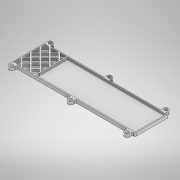
# Autodesk Inventor part: backtpackCOVER2
Saved by Autodesk Inventor 2021 (Build 250183000, 183)
## iProperties
Created: 2021-09-03
Part Number: backtpackCOVER2
Material: Generic
Document SubType Name: Modeling
Designer: perez
Density: 1 g/cm^3
Appearance: Default
Author: perez
Autodesk Inventor part; units mm, degrees
ref_plane "YZ Plane" through (0, 0, 0) normal (1, 0, 0) x (0, 1, 0)
ref_plane "XZ Plane" through (0, 0, 0) normal (0, 1, 0) x (-1, 0, 0)
ref_plane "XY Plane" through (0, 0, 0) normal (0, 0, 1) x (1, 0, 0)
sketch "Sketch1" plane through (0, 0, 0) normal (0, 1, 0) x (-1, 0, 0)
  line L0 (0, 0) -> (37, 0) construction
  line L1 (37, 0) -> (37, -30) construction
  line L2 (37, -30) -> (0, -30) construction
  line L3 (0, -30) -> (0, 0) construction
  line L4 (75.5, -6) -> (38, -6) construction
  line L5 (38, -6) -> (38, -24) construction
  line L6 (38, -24) -> (75.5, -24) construction
  line L7 (75.5, -24) -> (75.5, -6) construction
  line L8 (94, 0) -> (76.5, 0) construction
  line L9 (76.5, 0) -> (76.5, -28) construction
  line L10 (76.5, -28) -> (94, -28) construction
  line L11 (94, -28) -> (94, 0) construction
  line L12 (-1, 1) -> (117.5, 1)
  line L13 (117.5, 1) -> (117.5, -31)
  line L14 (117.5, -31) -> (-1, -31)
  line L15 (-1, -31) -> (-1, 1)
  line L16 (0, 0) -> (94, 0)
  line L17 (94, 0) -> (94, -30)
  line L18 (94, -30) -> (0, -30)
  line L19 (0, -30) -> (0, 0)
  line L20 (38, -8) -> (37, -8)
  line L21 (37, -8) -> (37, -22)
  line L22 (37, -22) -> (38, -22)
  line L23 (38, -22) -> (38, -8)
  line L24 (73.5, -6) -> (40, -6)
  line L25 (40, -6) -> (40, -5)
  line L26 (40, -5) -> (73.5, -5)
  line L27 (73.5, -5) -> (73.5, -6)
  line L28 (73.5, -24) -> (40, -24)
  line L29 (40, -24) -> (40, -25)
  line L30 (40, -25) -> (73.5, -25)
  line L31 (73.5, -25) -> (73.5, -24)
  line L32 (76.5, -8) -> (75.5, -8)
  line L33 (75.5, -8) -> (75.5, -22)
  line L34 (75.5, -22) -> (76.5, -22)
  line L35 (76.5, -22) -> (76.5, -8)
  line L36 (115, -31) -> (115, -33.5) construction
  line L37 (58.25, -31) -> (58.25, -33.5) construction
  line L38 (4, -31) -> (4, -33.5) construction
  line L39 (115, 1) -> (115, 3.5) construction
  line L40 (58.25, 1) -> (58.25, 3.5) construction
  line L41 (4, 1) -> (4, 3.5) construction
  circle A0 centre (115, -33.5) radius 2.5
  circle A1 centre (58.25, -33.5) radius 2.5
  circle A2 centre (4, -33.5) radius 2.5
  circle A3 centre (4, 3.5) radius 2.5
  circle A4 centre (58.25, 3.5) radius 2.5
  circle A5 centre (115, 3.5) radius 2.5
  line L42 (117.5, 1) -> (117.5, 3.5)
  line L43 (112.5, 3.5) -> (112.5, 1)
  line L44 (60.75, 3.5) -> (60.75, 1)
  line L45 (55.75, 3.5) -> (55.75, 1)
  line L46 (6.5, 3.5) -> (6.5, 1)
  line L47 (1.5, 3.5) -> (1.5, 1)
  line L48 (1.5, -33.5) -> (1.5, -31)
  line L49 (6.5, -33.5) -> (6.5, -31)
  line L50 (55.75, -33.5) -> (55.75, -31)
  line L51 (60.75, -33.5) -> (60.75, -31)
  line L52 (117.5, -33.5) -> (117.5, -31)
  line L53 (112.5, -33.5) -> (112.5, -31)
  circle A6 centre (115, -33.5) radius 1.55
  circle A7 centre (58.25, -33.5) radius 1.55
  circle A8 centre (4, -33.5) radius 1.55
  circle A9 centre (4, 3.5) radius 1.55
  circle A10 centre (58.25, 3.5) radius 1.55
  circle A11 centre (115, 3.5) radius 1.55
  line L54 (57.75, -30) -> (58.75, -30)
  line L55 (58.75, -30) -> (58.75, -25)
  line L56 (58.75, -25) -> (57.75, -25)
  line L57 (57.75, -25) -> (57.75, -30)
  line L58 (57.75, -5) -> (58.75, -5)
  line L59 (58.75, -5) -> (58.75, 0)
  line L60 (58.75, 0) -> (57.75, 0)
  line L61 (57.75, 0) -> (57.75, -5)
  line L62 (40, -25) -> (41, -25)
  line L63 (41, -25) -> (41, -30)
  line L64 (41, -30) -> (40, -30)
  line L65 (40, -30) -> (40, -25)
  line L66 (40, -5) -> (41, -5)
  line L67 (41, -5) -> (41, 0)
  line L68 (41, 0) -> (40, 0)
  line L69 (40, 0) -> (40, -5)
  line L70 (73.5, -5) -> (72.5, -5)
  line L71 (72.5, -5) -> (72.5, 0)
  line L72 (72.5, 0) -> (73.5, 0)
  line L73 (73.5, 0) -> (73.5, -5)
  line L74 (73.5, -25) -> (72.5, -25)
  line L75 (72.5, -25) -> (72.5, -30)
  line L76 (72.5, -30) -> (73.5, -30)
  line L77 (73.5, -30) -> (73.5, -25)
  dimension "d0" = 37
  dimension "d1" = 30
  dimension "d2" = 18
  dimension "d3" = 37.5
  dimension "d4" = 1
  dimension "d5" = 6
  dimension "d6" = 17.5
  dimension "d7" = 28
  dimension "d8" = 1
  dimension "d9" = 1
  dimension "d10" = 1
  dimension "d11" = 1
  dimension "d12" = 117.5
  dimension "d13" = 2
  dimension "d14" = 2
  dimension "d15" = 1
  dimension "d16" = 1
  dimension "d17" = 2
  dimension "d18" = 2
  dimension "d19" = 2
  dimension "d20" = 2
  dimension "d21" = 2.5
  dimension "d22" = 2.5
  dimension "d23" = 5
  dimension "d24" = 2.5
  dimension "d25" = 2.5
  dimension "d26" = 2.5
  dimension "d27" = 2.5
  dimension "d28" = 5
  dimension "d29" = 5
  dimension "d30" = 2.5
  dimension "d31" = 3.1
  dimension "d32" = 3.1
  dimension "d33" = 3.1
  dimension "d34" = 3.1
  dimension "d35" = 3.1
  dimension "d36" = 3.1
  dimension "d44" = 1
  dimension "d45" = 1
  dimension "d46" = 0.5
  dimension "d47" = 0
  dimension "d48" = 1
  dimension "d49" = 1
  dimension "d50" = 1
  dimension "d51" = 1
  constraints: 152 end point, 30 parallel, 24 point on line, 16 point on circle, 15 perpendicular, 14 horizontal, 12 centre point, 12 coincident, 12 vertical, 8 tangent, 22 other
  measures "d0" distance of L1.end L2.end
  measures "d1" distance of L0.end L1.end
  measures "d2" distance of L4.end L5.end
  measures "d3" distance of L5.end L6.end
  measures "d4" distance between parallel lines of L1 L5
  measures "d5" distance between parallel lines of L2 L6
  measures "d6" distance of L10.end L9.end
  measures "d7" distance of L9.end L8.end
  measures "d8" distance between parallel lines of L7 L9
  measures "d9" distance between parallel lines of L15 L3
  measures "d12" distance between parallel lines of L13 L3
  measures "d13" distance between parallel lines of L20 L4
  measures "d14" distance between parallel lines of L22 L6
  measures "d15" distance of L30.end L28.start
  measures "d16" distance of L26.end L24.start
  measures "d17" distance between parallel lines of L5 L25
  measures "d18" distance between parallel lines of L7 L27
  measures "d19" distance between parallel lines of L6 L34
  measures "d20" distance between parallel lines of L4 L32
  measures "d21" distance of L36.start L36.end
  measures "d22" distance between parallel lines of L13 L36
  measures "d23" distance between parallel lines of L15 L38
  measures "d24" distance of L37.start L37.end
  measures "d25" distance of L39.start L39.end
  measures "d26" distance of L40.start L40.end
  measures "d27" distance of L41.start L41.end
  measures "d28" diameter of A0
  measures "d29" diameter of A1
  measures "d30" distance of L38.start L38.end
  measures "d31" diameter of A6
  measures "d32" diameter of A7
  measures "d33" diameter of A8
  measures "d34" diameter of A9
  measures "d35" diameter of A10
  measures "d36" diameter of A11
  measures "d44" distance between parallel lines of L55 L57
  measures "d45" distance between parallel lines of L59 L61
  measures "d46" distance between parallel lines of L37 L57
  measures "d47" distance between parallel lines of L40 L37
  measures "d48" distance of L63.end L64.end
  measures "d49" distance of L68.end L67.end
  measures "d50" distance of L71.end L72.end
  measures "d51" distance of L76.end L75.end
extrude "Extrusion1" add sketch "Sketch1" along normal blind 7 contours L12 L13 L14 L15 | L47 A3 L12 | A3 L46 L12 | A3 | L14 A2 L48 | L14 L49 A2 | A2 | L45 A4 L12 | A4 L44 L12 | A4 | L14 A1 L50 | L14 L51 A1 | A1 | L43 A5 L12 | A5 L42 L12 | A5 | L14 A0 L53 | L14 L52 A0 | A0 | L16 L67 L26 L69 | L26 L27 L24 L25 | L65 L30 L63 L18 | L16 L59 L26 L61 | L29 L28 L31 L30 | L57 L30 L55 L18 | L16 L73 L26 L71 | L75 L30 L77 L18 | L23 L22 L21 L20 | L35 L34 L33 L32
sketch "Sketch2" plane through (0, 0, 0) normal (0, -1, 0) x (1, 0, 0)
  line L0 (-117.5, -33.5) -> (-117.5, 3.5) projected
  arc A0 (-117.5, -33.5) -> (-112.5, -33.5) centre (-115, -33.5) ccw projected
  line L1 (-112.5, -31) -> (-112.5, -33.5) projected
  line L2 (-60.75, -31) -> (-112.5, -31) projected
  line L3 (-60.75, -33.5) -> (-60.75, -31) projected
  arc A1 (-60.75, -33.5) -> (-55.75, -33.5) centre (-58.25, -33.5) ccw projected
  line L4 (-55.75, -31) -> (-55.75, -33.5) projected
  line L5 (-6.5, -31) -> (-55.75, -31) projected
  line L6 (-6.5, -33.5) -> (-6.5, -31) projected
  arc A2 (-6.5, -33.5) -> (-1.5, -33.5) centre (-4, -33.5) ccw projected
  line L7 (-1.5, -31) -> (-1.5, -33.5) projected
  line L8 (1, -31) -> (-1.5, -31) projected
  line L9 (1, 1) -> (1, -31) projected
  line L10 (-1.5, 1) -> (1, 1) projected
  line L11 (-1.5, 3.5) -> (-1.5, 1) projected
  arc A3 (-1.5, 3.5) -> (-6.5, 3.5) centre (-4, 3.5) ccw projected
  line L12 (-6.5, 1) -> (-6.5, 3.5) projected
  line L13 (-55.75, 1) -> (-6.5, 1) projected
  line L14 (-55.75, 3.5) -> (-55.75, 1) projected
  arc A4 (-55.75, 3.5) -> (-60.75, 3.5) centre (-58.25, 3.5) ccw projected
  line L15 (-60.75, 1) -> (-60.75, 3.5) projected
  line L16 (-112.5, 1) -> (-60.75, 1) projected
  line L17 (-112.5, 3.5) -> (-112.5, 1) projected
  arc A5 (-112.5, 3.5) -> (-117.5, 3.5) centre (-115, 3.5) ccw projected
  circle A6 centre (-58.25, 3.5) radius 1.55 projected
  circle A7 centre (-4, 3.5) radius 1.55 projected
  circle A8 centre (-4, -33.5) radius 1.55 projected
  circle A9 centre (-58.25, -33.5) radius 1.55 projected
  circle A10 centre (-115, 3.5) radius 1.55 projected
  circle A11 centre (-115, -33.5) radius 1.55 projected
  line L18 (-41, 0) -> (-57.75, 0) projected
  line L19 (0, -30) -> (0, 0) projected
  line L20 (-57.75, -30) -> (-41, -30) projected
  line L21 (-94, 0) -> (-94, -30) projected
  line L22 (-41, -5) -> (-41, 0) projected
  line L23 (-57.75, -5) -> (-41, -5) projected
  line L24 (-57.75, 0) -> (-57.75, -5) projected
  line L25 (-41, -30) -> (-41, -25) projected
  line L26 (-57.75, -25) -> (-57.75, -30) projected
  line L27 (-41, -25) -> (-57.75, -25) projected
  line L28 (-72.5, -25) -> (-72.5, -30) projected
  line L29 (-58.75, -25) -> (-72.5, -25) projected
  line L30 (-58.75, -30) -> (-58.75, -25) projected
  line L31 (-72.5, -30) -> (-58.75, -30) projected
  line L32 (-72.5, 0) -> (-72.5, -5) projected
  line L33 (-58.75, 0) -> (-72.5, 0) projected
  line L34 (-58.75, -5) -> (-58.75, 0) projected
  line L35 (-72.5, -5) -> (-58.75, -5) projected
  line L36 (-73.5, 0) -> (-94, 0) projected
  line L37 (-73.5, -6) -> (-73.5, 0) projected
  line L38 (-40, -6) -> (-73.5, -6) projected
  line L39 (-40, 0) -> (-40, -6) projected
  line L40 (0, 0) -> (-40, 0) projected
  line L41 (-40, -30) -> (0, -30) projected
  line L42 (-40, -24) -> (-40, -30) projected
  line L43 (-73.5, -24) -> (-40, -24) projected
  line L44 (-73.5, -30) -> (-73.5, -24) projected
  line L45 (-94, -30) -> (-73.5, -30) projected
extrude "Extrusion2" add sketch "Sketch2" along normal blind 1 contours L0 A5 L17 L16 L15 A4 L14 L13 L12 A3 L11 L10 L9 L8 L7 A2 L6 L5 L4 A1 L3 L2 L1 A0 | L22 L23 L24 L18 | L41 L42 L43 L44 L45 L21 L36 L37 L38 L39 L40 L19 | L26 L27 L25 L20 | L29 L30 L31 L28 | L33 L34 L35 L32
fillet "Fillet2" radius 1 32 edges at (-73.5, 3.5, -6) (-73.5, 3.5, -24) (-40, 3.5, -24) (1, 3, -31) (-1.5, 3, -31) (1, 3, 1) (-55.75, 3, -31) (-1.5, 3, 1) (-55.75, 3, 1) (-112.5, 3, 1) (-112.5, 3, -31) (-60.75, 3, -31) (-6.5, 3, -31) (-60.75, 3, 1) (-6.5, 3, 1) (-40, 3.5, -6) (-72.5, 3.5, 0) (-57.75, 3.5, 0) (-72.5, 3.5, -25) (-57.75, 3.5, -25) (-41, 3.5, -25) (-58.75, 3.5, -25) (-41, 3.5, 0) (-58.75, 3.5, 0) (-72.5, 3.5, -30) (-57.75, 3.5, -30) (-57.75, 3.5, -5) (-72.5, 3.5, -5) (-41, 3.5, -5) (-58.75, 3.5, -5) (-58.75, 3.5, -30) (-41, 3.5, -30)
sketch "Sketch5" plane through (0, 7, 0) normal (0, 1, 0) x (1, 0, 0)
  line L0 (-120.447, 38.9055) -> (3.6698, 38.9055)
  line L1 (3.6698, 38.9055) -> (3.6698, -10.7705)
  line L2 (3.6698, -10.7705) -> (-120.447, -10.7705)
  line L3 (-120.447, -10.7705) -> (-120.447, 38.9055)
  point P0 (0, 0)
  constraints: 8 end point, 2 parallel, 1 horizontal, 1 perpendicular
extrude "Extrusion5" cut sketch "Sketch5" against normal blind 7
sketch "Sketch14" plane through (0, 0, 0) normal (0, 1, 0) x (1, 0, 0)
  line L0 (0, 30) -> (-95, 30)
  line L1 (-95, 30) -> (-95, 0)
  line L2 (-95, 0) -> (0, 0)
  line L3 (0, 0) -> (0, 30)
  line L4 (-54.75, 31) -> (-7.5, 31) projected
  line L5 (1, 30) -> (1, 0) projected
  line L6 (-7.5, -1) -> (-54.75, -1) projected
  line L7 (-117.5, -3.5) -> (-117.5, 33.5) projected
  circle A0 centre (-58.25, -3.5) radius 1.55 projected
  circle A1 centre (-4, -3.5) radius 1.55 projected
  circle A2 centre (-4, 33.5) radius 1.55 projected
  circle A3 centre (-58.25, 33.5) radius 1.55 projected
  circle A4 centre (-115, -3.5) radius 1.55 projected
  circle A5 centre (-115, 33.5) radius 1.55 projected
  arc A6 (1, 30) -> (0, 31) centre (0, 30) ccw projected
  line L8 (-0.5, 31) -> (0, 31) projected
  arc A7 (-1.5, 32) -> (-0.5, 31) centre (-0.5, 32) ccw projected
  line L9 (-1.5, 33.5) -> (-1.5, 32) projected
  arc A8 (-1.5, 33.5) -> (-6.5, 33.5) centre (-4, 33.5) ccw projected
  line L10 (-6.5, 32) -> (-6.5, 33.5) projected
  arc A9 (-7.5, 31) -> (-6.5, 32) centre (-7.5, 32) ccw projected
  line L11 (-54.75, 31) -> (-7.5, 31) projected
  arc A10 (-55.75, 32) -> (-54.75, 31) centre (-54.75, 32) ccw projected
  line L12 (-55.75, 33.5) -> (-55.75, 32) projected
  arc A11 (-55.75, 33.5) -> (-60.75, 33.5) centre (-58.25, 33.5) ccw projected
  line L13 (-60.75, 32) -> (-60.75, 33.5) projected
  arc A12 (-61.75, 31) -> (-60.75, 32) centre (-61.75, 32) ccw projected
  line L14 (-111.5, 31) -> (-61.75, 31) projected
  arc A13 (-112.5, 32) -> (-111.5, 31) centre (-111.5, 32) ccw projected
  line L15 (-112.5, 33.5) -> (-112.5, 32) projected
  arc A14 (-112.5, 33.5) -> (-117.5, 33.5) centre (-115, 33.5) ccw projected
  line L16 (-117.5, -3.5) -> (-117.5, 33.5) projected
  arc A15 (-117.5, -3.5) -> (-112.5, -3.5) centre (-115, -3.5) ccw projected
  line L17 (-112.5, -2) -> (-112.5, -3.5) projected
  arc A16 (-111.5, -1) -> (-112.5, -2) centre (-111.5, -2) ccw projected
  line L18 (-61.75, -1) -> (-111.5, -1) projected
  arc A17 (-60.75, -2) -> (-61.75, -1) centre (-61.75, -2) ccw projected
  line L19 (-60.75, -3.5) -> (-60.75, -2) projected
  arc A18 (-60.75, -3.5) -> (-55.75, -3.5) centre (-58.25, -3.5) ccw projected
  line L20 (-55.75, -2) -> (-55.75, -3.5) projected
  arc A19 (-54.75, -1) -> (-55.75, -2) centre (-54.75, -2) ccw projected
  line L21 (-7.5, -1) -> (-54.75, -1) projected
  arc A20 (-6.5, -2) -> (-7.5, -1) centre (-7.5, -2) ccw projected
  line L22 (-6.5, -3.5) -> (-6.5, -2) projected
  arc A21 (-6.5, -3.5) -> (-1.5, -3.5) centre (-4, -3.5) ccw projected
  line L23 (-1.5, -2) -> (-1.5, -3.5) projected
  arc A22 (-0.5, -1) -> (-1.5, -2) centre (-0.5, -2) ccw projected
  line L24 (0, -1) -> (-0.5, -1) projected
  arc A23 (0, -1) -> (1, 0) centre (0, 0) ccw projected
  line L25 (1, 30) -> (1, 0) projected
  line L26 (-116.5, 0) -> (-96.2679, 0)
  line L27 (-96.2679, 0) -> (-96.2679, 30)
  line L28 (-96.2679, 30) -> (-116.5, 30)
  line L29 (-116.5, 30) -> (-116.5, 0)
  line L30 (-120.0355, 30) -> (-116.5, 33.5355)
  line L31 (-116.5, 33.5355) -> (-112.9645, 30)
  line L32 (-112.9645, 30) -> (-116.5, 26.4645)
  line L33 (-116.5, 26.4645) -> (-120.0355, 30)
  line L34 (-115.6376, 25.602) -> (-112.102, 22.0665)
  line L35 (-112.102, 22.0665) -> (-108.5665, 25.602)
  line L36 (-108.5665, 25.602) -> (-112.102, 29.1376)
  line L37 (-112.102, 29.1376) -> (-115.6376, 25.602)
  line L38 (-111.0355, 30) -> (-107.5, 33.5355)
  line L39 (-107.5, 26.4645) -> (-111.0355, 30)
  line L40 (-103.9645, 30) -> (-107.5, 26.4645)
  line L41 (-107.5, 33.5355) -> (-103.9645, 30)
  line L42 (-99.5665, 25.602) -> (-103.102, 29.1376)
  line L43 (-103.102, 29.1376) -> (-106.6376, 25.602)
  line L44 (-106.6376, 25.602) -> (-103.102, 22.0665)
  line L45 (-103.102, 22.0665) -> (-99.5665, 25.602)
  line L46 (-102.0355, 30) -> (-98.5, 33.5355)
  line L47 (-98.5, 26.4645) -> (-102.0355, 30)
  line L48 (-94.9645, 30) -> (-98.5, 26.4645)
  line L49 (-98.5, 33.5355) -> (-94.9645, 30)
  line L50 (-90.5665, 25.602) -> (-94.102, 29.1376)
  line L51 (-94.102, 29.1376) -> (-97.6376, 25.602)
  line L52 (-97.6376, 25.602) -> (-94.102, 22.0665)
  line L53 (-94.102, 22.0665) -> (-90.5665, 25.602)
  line L54 (-120.0355, 21) -> (-116.5, 24.5355)
  line L55 (-116.5, 17.4645) -> (-120.0355, 21)
  line L56 (-112.9645, 21) -> (-116.5, 17.4645)
  line L57 (-116.5, 24.5355) -> (-112.9645, 21)
  line L58 (-108.5665, 16.602) -> (-112.102, 20.1376)
  line L59 (-112.102, 20.1376) -> (-115.6376, 16.602)
  line L60 (-115.6376, 16.602) -> (-112.102, 13.0665)
  line L61 (-112.102, 13.0665) -> (-108.5665, 16.602)
  line L62 (-111.0355, 21) -> (-107.5, 24.5355)
  line L63 (-107.5, 17.4645) -> (-111.0355, 21)
  line L64 (-103.9645, 21) -> (-107.5, 17.4645)
  line L65 (-107.5, 24.5355) -> (-103.9645, 21)
  line L66 (-99.5665, 16.602) -> (-103.102, 20.1376)
  line L67 (-103.102, 20.1376) -> (-106.6376, 16.602)
  line L68 (-106.6376, 16.602) -> (-103.102, 13.0665)
  line L69 (-103.102, 13.0665) -> (-99.5665, 16.602)
  line L70 (-102.0355, 21) -> (-98.5, 24.5355)
  line L71 (-98.5, 17.4645) -> (-102.0355, 21)
  line L72 (-94.9645, 21) -> (-98.5, 17.4645)
  line L73 (-98.5, 24.5355) -> (-94.9645, 21)
  line L74 (-90.5665, 16.602) -> (-94.102, 20.1376)
  line L75 (-94.102, 20.1376) -> (-97.6376, 16.602)
  line L76 (-97.6376, 16.602) -> (-94.102, 13.0665)
  line L77 (-94.102, 13.0665) -> (-90.5665, 16.602)
  line L78 (-120.0355, 12) -> (-116.5, 15.5355)
  line L79 (-116.5, 8.4645) -> (-120.0355, 12)
  line L80 (-112.9645, 12) -> (-116.5, 8.4645)
  line L81 (-116.5, 15.5355) -> (-112.9645, 12)
  line L82 (-108.5665, 7.602) -> (-112.102, 11.1376)
  line L83 (-112.102, 11.1376) -> (-115.6376, 7.602)
  line L84 (-115.6376, 7.602) -> (-112.102, 4.0665)
  line L85 (-112.102, 4.0665) -> (-108.5665, 7.602)
  line L86 (-111.0355, 12) -> (-107.5, 15.5355)
  line L87 (-107.5, 8.4645) -> (-111.0355, 12)
  line L88 (-103.9645, 12) -> (-107.5, 8.4645)
  line L89 (-107.5, 15.5355) -> (-103.9645, 12)
  line L90 (-99.5665, 7.602) -> (-103.102, 11.1376)
  line L91 (-103.102, 11.1376) -> (-106.6376, 7.602)
  line L92 (-106.6376, 7.602) -> (-103.102, 4.0665)
  line L93 (-103.102, 4.0665) -> (-99.5665, 7.602)
  line L94 (-102.0355, 12) -> (-98.5, 15.5355)
  line L95 (-98.5, 8.4645) -> (-102.0355, 12)
  line L96 (-94.9645, 12) -> (-98.5, 8.4645)
  line L97 (-98.5, 15.5355) -> (-94.9645, 12)
  line L98 (-90.5665, 7.602) -> (-94.102, 11.1376)
  line L99 (-94.102, 11.1376) -> (-97.6376, 7.602)
  line L100 (-97.6376, 7.602) -> (-94.102, 4.0665)
  line L101 (-94.102, 4.0665) -> (-90.5665, 7.602)
  line L102 (-120.0355, 3) -> (-116.5, 6.5355)
  line L103 (-116.5, -0.5355) -> (-120.0355, 3)
  line L104 (-112.9645, 3) -> (-116.5, -0.5355)
  line L105 (-116.5, 6.5355) -> (-112.9645, 3)
  line L106 (-108.5665, -1.398) -> (-112.102, 2.1376)
  line L107 (-112.102, 2.1376) -> (-115.6376, -1.398)
  line L108 (-115.6376, -1.398) -> (-112.102, -4.9335)
  line L109 (-112.102, -4.9335) -> (-108.5665, -1.398)
  line L110 (-111.0355, 3) -> (-107.5, 6.5355)
  line L111 (-107.5, -0.5355) -> (-111.0355, 3)
  line L112 (-103.9645, 3) -> (-107.5, -0.5355)
  line L113 (-107.5, 6.5355) -> (-103.9645, 3)
  line L114 (-99.5665, -1.398) -> (-103.102, 2.1376)
  line L115 (-103.102, 2.1376) -> (-106.6376, -1.398)
  line L116 (-106.6376, -1.398) -> (-103.102, -4.9335)
  line L117 (-103.102, -4.9335) -> (-99.5665, -1.398)
  line L118 (-102.0355, 3) -> (-98.5, 6.5355)
  line L119 (-98.5, -0.5355) -> (-102.0355, 3)
  line L120 (-94.9645, 3) -> (-98.5, -0.5355)
  line L121 (-98.5, 6.5355) -> (-94.9645, 3)
  line L122 (-90.5665, -1.398) -> (-94.102, 2.1376)
  line L123 (-94.102, 2.1376) -> (-97.6376, -1.398)
  line L124 (-97.6376, -1.398) -> (-94.102, -4.9335)
  line L125 (-94.102, -4.9335) -> (-90.5665, -1.398)
  point P0 (0, 0)
  point P1 (-7.5, 31)
  point P2 (1, 0)
  point P3 (-112.6588, -4.3768)
  point P4 (-108.9645, -1)
  point P5 (-96.2679, 28.6966)
  point P6 (-95, 2.9645)
  point P7 (-95, 3.0355)
  point P8 (-96.2679, 22.3034)
  point P9 (-96.2679, 19.6966)
  point P10 (-96.2679, 17.9717)
  point P11 (-96.2679, 15.2323)
  point P12 (-96.2679, 13.3034)
  point P13 (-96.2679, 10.6966)
  point P14 (-96.2679, 8.9717)
  point P15 (-96.2679, 6.2323)
  point P16 (-100.9645, 0)
  point P17 (-105.2396, 0)
  point P18 (-96.2679, 1.6966)
  point P19 (-97.9645, 0)
  point P20 (-99.0355, 0)
  point P21 (-96.2679, 4.3034)
  point P22 (-108.0355, 0)
  point P23 (-106.9645, 0)
  point P24 (-109.9645, 0)
  point P25 (-114.2396, 0)
  point P26 (-115.9645, 0)
  point P27 (-113.4522, -3.5833)
  point P28 (-115.0833, -1.9522)
  point P29 (-96.2679, 26.9717)
  point P30 (-96.2679, 24.2323)
  dimension "d127" = 1
  dimension "d128" = 1
  dimension "d129" = 1
  dimension "d130" = 22.5
  dimension "d133" = 1
  dimension "d134" = 1
  dimension "d135" = 1
  dimension "d136" = 5
  dimension "d137" = 5
  dimension "d138" = 0
  dimension "d139" = 0
  dimension "d140" = 5
  dimension "d141" = 5
  dimension "d144" = 9
  dimension "d147" = 9
  constraints: 208 end point, 6 parallel, 5 perpendicular, 3 horizontal, 1 vertical, 176 other
  measures "d127" distance between parallel lines of L0 L4
  measures "d128" distance between parallel lines of L3 L5
  measures "d129" distance between parallel lines of L6 L2
  measures "d130" distance between parallel lines of L7 L1
  measures "d133" distance between parallel lines of L7 L29
  measures "d134" distance between parallel lines of L14 L28
  measures "d135" distance between parallel lines of L18 L26
  measures "d136" distance of L30.start L30.end
  measures "d137" distance of L30.end L31.end
  measures "d138" distance from line of L0 L31.end
  measures "d139" distance from line of L29 L32.end
  measures "d140" distance between parallel lines of L34 L36
  measures "d141" distance between parallel lines of L35 L37
  measures "d144" distance of L30.start L38.start
  measures "d147" distance of L30.start L54.start
extrude "Extrusion16" add sketch "Sketch14" along normal blind 2 contours L0 L49 L14 A12 L13 A11 L12 A10 L4 A9 L10 A8 L9 A7 L8 A6 L5 A23 L24 A22 L23 A21 L22 A20 L6 A19 L20 A18 L19 A17 L18 L122 L2 L3 | L0 L1 L48 L27 L28 L46 L14 L49 | L1 L51 L27 L48 | L122 L18 L123 L1 L2 | L1 L52 L27 L51 | L27 L51 L52 L73 L70 L71 L72 L75 L76 L97 L94 L95 L96 L99 L100 L121 L118 L119 L26 L114 L115 L112 L113 L110 L111 L106 L107 L104 L105 L29 L80 L81 L56 L57 L32 L28 L39 L40 L47 L48 | L46 L28 L41 L14 | L1 L73 L27 L52 | L41 L28 L38 L14 | L123 L18 L114 L26 L119 L120 L27 L1 | L1 L72 L27 L73 | L38 L28 L31 A5 L30 L7 A14 L15 A13 L14 | L120 L27 L121 L1 | L1 L121 L120 | L18 L115 L26 L114 | L1 L75 L27 L72 | L121 L27 L100 L1 | L27 L26 L120 | L18 L106 L26 L111 L112 L115 | L1 L76 L27 L75 | L28 L29 L33 L7 L30 A5 L31 | L100 L27 L99 L1 | L120 L119 L26 | L18 A16 L17 A15 L108 A4 L107 L26 L106 | L1 L97 L27 L76 | L29 L54 L7 L33 | L99 L27 L96 L1 | L112 L111 L26 | L1 L96 L27 L97 | L29 L55 L7 L54 | L107 L108 A4 A15 L7 L103 L104 L26 | L29 L78 L7 L55 | L104 L103 L7 L102 L29 L26 | L29 L79 L7 L78 | L29 L102 L7 L79
body "Solid1"
